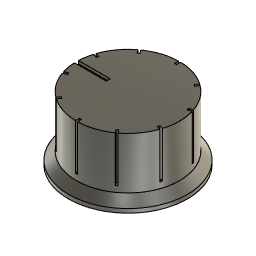
Knob (Autodesk Fusion 360 design; units mm, degrees)
Autodesk Fusion 360 part; units mm, degrees
sketch "Sketch1" plane through (0, 0, 0) normal (0, 0, 1) x (1, 0, 0) in component "Knob"
  circle A0 centre (0, 0) radius 15
  dimension "d1" = 30
  constraint coincident A0.centre origin
  measures "d1" diameter of A0
extrude "Extrude1" add sketch "Sketch1" along normal blind 3 makes body 1 in component "Knob"
sketch "Sketch2" plane through (0, 0, 3) normal (0, 0, 1) x (-1, 0, 0) in component "Knob"
  circle A0 centre (0, 0) radius 15
  circle A1 centre (0, 0) radius 13
  dimension "d7" = 26
  measures "d7" diameter of A1
extrude "Extrude2" add sketch "Sketch2" along normal blind 13 separate body contours A1 makes body 2 in component "Knob"
hole "Hole2" at (0, 0, 3) direction (0, 0, 1) diameter 6.1 depth 12 tip angle 180 bodies 2 in component "Knob"
sketch "Sketch5" plane through (0, 0, 0) normal (0, 1, 0) x (1, 0, 0) in component "Knob"
  line L0 (0, -3) -> (0, 0)
  line L1 (0, 0) -> (10, 0)
  line L2 (10, 0) -> (10, -3)
  line L3 (10, -3) -> (0, -3)
  dimension "d26" = 10
  dimension "d27" = 3
  constraint coincident L0.end L1.start
  constraint vertical L0
  constraint perpendicular L0 L1
  constraint perpendicular L1 L2
  constraint perpendicular L0 L3
  measures "d26" distance of L0.end L1.end
  measures "d27" distance of L1.end L2.end
revolve "Revolve1" cut sketch "Sketch5" angle 360 about axis through (0, 0, 3) along (0, 0, -1) bodies 1 in component "Knob"
sketch "Sketch6" plane through (0, 0, 16) normal (0, 0, 1) x (-1, 0, 0) in component "Knob"
  line L0 (5, -0.5) -> (15, -0.5)
  line L1 (15, -0.5) -> (15, 0.5)
  line L2 (15, 0.5) -> (5, 0.5)
  line L3 (5, 0.5) -> (5, -0.5)
  circle A0 centre (0, 0) radius 13
  dimension "d29" = 5
  dimension "d30" = 10
  dimension "d31" = 1
  dimension "d32" = 0.5
  constraint horizontal L0
  constraint vertical L1
  constraint horizontal L2
  constraint vertical L3
  measures "d29" distance of A0.centre L3
  measures "d30" distance of L0.start L0.end
  measures "d31" distance of L0.end L1.end
  measures "d32" distance of A0.centre L0
extrude "Extrude3" cut sketch "Sketch6" against normal blind 1 contours L0 L2 L3 A0 | L0 L1 L2 A0 picked at (7.6667, 0) bodies 2 in component "Knob"
chamfer "Chamfer2" distance 0.3 angle 45 2 edges at (-8.9952, 0.5, 15) (-8.9952, -0.5, 15) on bodies 2 in component "Knob"
sketch "Sketch1 (2)" plane through (0, 0, 16) normal (0, 0, 1) x (-1, 0, 0)
  line L0 (5, -0.5) -> (5, 0.5)
  line L1 (0.25, -13.5) -> (-0.25, -13.5)
  line L2 (-0.25, -13.5) -> (-0.25, -12)
  line L3 (-0.25, -12) -> (0.25, -12)
  line L4 (0.25, -12) -> (0.25, -13.5)
  arc A0 (12.9904, 0.5) -> (12.9904, -0.5) centre (0, 0) ccw
  line L5 (12.9904, -0.5) -> (5, -0.5)
  line L6 (5, 0.5) -> (12.9904, 0.5)
  dimension "d36" = 0.5
  dimension "d37" = 1.5
  dimension "d38" = 0.25
  dimension "d39" = 13.5
  constraint horizontal L1
  constraint vertical L2
  constraint horizontal L3
  constraint vertical L4
  measures "d36" distance of L1.start L1.end
  measures "d37" distance of L1.end L2.end
  measures "d38" horizontal distance of A0.centre L2.end
  measures "d39" distance of A0.centre L1
extrude "Extrude4" cut sketch "Sketch1 (2)" against normal blind 11.5 contours L2 L3 L4 A0 | L1 L2 L4 A0 bodies 2 in component "Knob"
chamfer "Chamfer4" distance 2 angle 45 1 edges at (-13.9849, -5.4242, 3) on bodies 1 in component "Knob"
chamfer "Chamfer6" distance 0.5 angle 45 1 edges at (0, 12, 4.5) on bodies 2 in component "Knob"
pattern_circular "C-Pattern3" count 10 over 360 about axis through (0, 0, 16) along (0, 0, 1) of "Extrude4" in component "Knob"
sketch "Sketch2 (2)" plane through (0, 0, 15) normal (0, 0, -1) x (1, 0, 0)
  circle A0 centre (0, 0) radius 3.05
  line L0 (-0.4, 3.1) -> (0.4, 3.1)
  line L1 (0.4, 3.1) -> (0.4, -3.1)
  line L2 (0.4, -3.1) -> (-0.4, -3.1)
  line L3 (-0.4, -3.1) -> (-0.4, 3.1)
  line L4 (0, 3.1) -> (0, -3.1) construction
  dimension "d50" = 6.2
  dimension "d51" = 0.8
  constraint horizontal L0
  constraint vertical L1
  constraint horizontal L2
  constraint vertical L3
  constraint midpoint L0 L4.start
  constraint midpoint L2 L4.end
  constraint midpoint A0.centre L4
  measures "d50" distance of L0.end L1.end
  measures "d51" distance of L1 L3
extrude "Extrude5" add sketch "Sketch2 (2)" along normal blind 10 contours A0 L1 L3 | A0 L0 L1 L3 | A0 L1 L2 L3 bodies 2 in component "Knob"
component "Knob" placed x (1, 0, 0) y (0, 1, 0) z (0, 0, 1) at (0, 0, 0)
